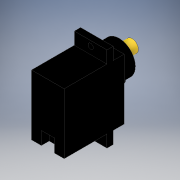
# Autodesk Inventor part: microservo_FT
Saved by Autodesk Inventor 2018 (Build 220112000, 112)
## iProperties
Created: 2018-02-08
Part Number: microservo_FT
Material: Genérico
Document SubType Name: Modeling
Designer: se_ma
Density: 1 g/cm^3
Appearance: Valor por defecto
Author: se_ma
Autodesk Inventor part; units mm, degrees
ref_plane "YZ Plane" through (0, 0, 0) normal (1, 0, 0) x (0, 1, 0)
ref_plane "XZ Plane" through (0, 0, 0) normal (0, 1, 0) x (-1, 0, 0)
ref_plane "XY Plane" through (0, 0, 0) normal (0, 0, 1) x (1, 0, 0)
sketch "Boceto1" plane through (0, 0, 0) normal (0, 1, 0) x (-1, 0, 0)
  line L0 (0, 0) -> (11.8, 0)
  line L1 (11.8, 0) -> (11.8, -23.2)
  line L2 (11.8, -23.2) -> (0, -23.2)
  line L3 (0, -23.2) -> (0, 0)
  dimension "d0" = 11.8
  dimension "d1" = 23.2
  constraints: 8 end point, 2 parallel, 1 horizontal, 1 perpendicular
  measures "d0" distance of L1.end L2.end
  measures "d1" distance of L0.end L1.end
extrude "Extrusión1" add sketch "Boceto1" along normal blind 23
sketch "Boceto2" plane through (0, 0, 0) normal (1, 0, 0) x (0, 0, -1)
  line L0 (0, 0) -> (0, 23) projected
  line L1 (0, 0) -> (0, 16.4)
  line L2 (0, 16.4) -> (-4.7, 16.4)
  line L3 (-4.7, 16.4) -> (-4.7, 18.8)
  line L4 (-4.7, 18.8) -> (0, 18.8)
  line L5 (23.2, 0) -> (23.2, 23) projected
  line L6 (23.2, 16.4) -> (27.9, 16.4)
  line L7 (27.9, 16.4) -> (27.9, 18.8)
  line L8 (27.9, 18.8) -> (23.2, 18.8)
  line L9 (0, 18.8) -> (0, 16.4)
  line L10 (23.2, 18.8) -> (23.2, 16.4)
  dimension "d4" = 16.4
  dimension "d5" = 4.7
  dimension "d6" = 2.4
  dimension "d7" = 4.7
  constraints: 18 end point, 7 point on line, 3 perpendicular, 2 collinear, 1 parallel
  measures "d4" distance of L0.start L1.end
  measures "d5" distance of L1.end L2.end
  measures "d6" distance of L2.end L3.end
  measures "d7" distance of L6.start L6.end
extrude "Extrusión2" add sketch "Boceto2" against normal blind 11.8
move faces "Desplazar1" translate (0.7, 0, 0) faces at (0, 5.4667, -15.4667)
sketch "Boceto4" plane through (-11.8, 18.8, 4.7) normal (0, 1, 0) x (1, 0, 0)
  line L0 (12.5, 0) -> (12.5, 4.7) projected
  line L1 (0, 0) -> (12.5, 0)
  line L2 (12.5, 0) -> (0, 0) projected
  line L3 (6.25, 0) -> (6.25, 1.9)
  line L4 (0, 32.6) -> (0, 27.9) projected
  line L5 (12.5, 32.6) -> (0, 32.6) projected
  line L6 (0, 32.6) -> (12.5, 32.6)
  line L7 (6.25, 32.6) -> (6.25, 30.7)
  circle A0 centre (6.25, 1.9) radius 1
  circle A1 centre (6.25, 30.7) radius 1
  point P0 (11.8, 4.7)
  dimension "d13" = 1.9
  dimension "d14" = 1.9
  dimension "d15" = 2
  dimension "d16" = 2
  constraints: 8 end point, 2 centre point, 2 coincident, 2 horizontal, 2 midpoint, 2 vertical
  measures "d13" distance of L3.start L3.end
  measures "d14" distance of L7.start L7.end
  measures "d15" diameter of A0
  measures "d16" diameter of A1
extrude "Extrusión3" cut sketch "Boceto4" against normal blind 2.4
sketch "Boceto5" plane through (0, 23, 0) normal (0, 1, 0) x (1, 0, 0)
  line L0 (-11.8, 23.2) -> (-11.8, 0) projected
  line L1 (-11.8, 0) -> (0.7, 0) projected
  line L2 (-11.8, 0) -> (0.7, 0)
  line L3 (0.7, 0) -> (0.7, 15)
  line L4 (0.7, 0) -> (0.7, 23.2) projected
  line L5 (0.7, 15) -> (-11.8, 15)
  line L6 (-11.8, 15) -> (-11.8, 0)
  point P0 (0, 0)
  dimension "d19" = 15
  constraints: 8 end point, 2 perpendicular, 1 collinear, 1 point on line
  measures "d19" distance of L1.end L3.end
extrude "Extrusión4" add sketch "Boceto5" along normal blind 4.3
sketch "Boceto6" plane through (0, 27.3, 0) normal (0, 1, 0) x (1, 0, 0)
  line L0 (-11.8, 0) -> (0.7, 0) projected
  line L1 (-5.55, 0) -> (-5.55, 5)
  circle A0 centre (-5.55, 5) radius 2.4
  point P0 (0, 0)
  dimension "d22" = 5
  dimension "d23" = 4.8
  constraints: 2 end point, 1 centre point, 1 coincident, 1 midpoint, 1 vertical
  measures "d22" distance of L1.start L1.end
  measures "d23" diameter of A0
extrude "Extrusión5" add sketch "Boceto6" along normal blind 5
sketch "Boceto7" plane through (0, 27.3, 0) normal (0, 1, 0) x (1, 0, 0)
  line L0 (-11.8, 0) -> (0.7, 0) projected
  line L1 (-5.55, 0) -> (-5.55, 6.25)
  arc A0 (-7.9995, 12) -> (-3.1005, 12) centre (-5.55, 6.25) ccw
  line L2 (0.7, 15) -> (-11.8, 15) projected
  arc A1 (-3.1005, 12) -> (-7.9995, 12) centre (-5.55, 12.5) ccw
  line L3 (0.7, 0) -> (-11.8, 0)
  line L4 (-11.8, 15) -> (-11.8, 0) projected
  line L5 (-11.8, 0) -> (-11.8, 15)
  line L6 (-11.8, 15) -> (0.7, 15)
  line L7 (0.7, 23.2) -> (0.7, 0) projected
  line L8 (0.7, 0) -> (0.7, 15)
  point P0 (0, 0)
  dimension "d26" = 6.25
  constraints: 10 end point, 5 point on circle, 3 collinear, 2 centre point, 1 coincident, 1 midpoint, 1 perpendicular, 1 vertical
  measures "d26" distance of L1.start L1.end
extrude "Extrusión6" cut sketch "Boceto7" against normal blind 4.3 contours L4 A0 L0 | A0 L7 L0 | L4 L2 A1 A0 | A0 A1 L2 L7
sketch "Boceto8" plane through (-11.8, 0, -23.2) normal (0, 0, -1) x (-1, 0, 0)
  line L0 (-12.5, 0) -> (0, 0) projected
  line L1 (-12.5, 0) -> (0, 0)
  line L2 (-6.25, 0) -> (-6.25, 3)
  line L3 (-6.25, 3) -> (-8.75, 3)
  line L4 (-8.75, 3) -> (-8.75, 0)
  line L5 (-6.25, 3) -> (-3.75, 3)
  line L6 (-3.75, 3) -> (-3.75, 0)
  point P0 (-11.8, 0)
  dimension "d30" = 3
  dimension "d31" = 2.5
  dimension "d32" = 2.5
  constraints: 12 end point, 3 perpendicular, 2 point on line, 1 collinear, 1 horizontal, 1 midpoint, 1 vertical
  measures "d30" distance of L2.start L2.end
  measures "d31" distance of L2.end L3.end
  measures "d32" distance of L2.end L5.end
extrude "Extrusión7" cut sketch "Boceto8" against normal blind 5
